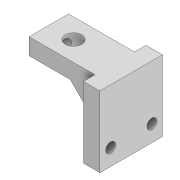
# Autodesk Inventor part: Mitutoyo holder
Saved by Autodesk Inventor 2020 (Build 240168000, 168)
## iProperties
Created: 2022-05-11
Part Number: Mitutoyo holder
Material: Generic
Document SubType Name: Modeling
Designer: ferrerx
Density: 1 g/cm^3
Appearance: Default
Author: ferrerx
Autodesk Inventor part; units mm, degrees
ref_plane "YZ Plane" through (0, 0, 0) normal (1, 0, 0) x (0, 1, 0)
ref_plane "XZ Plane" through (0, 0, 0) normal (0, 1, 0) x (-1, 0, 0)
ref_plane "XY Plane" through (0, 0, 0) normal (0, 0, 1) x (1, 0, 0)
sketch "Sketch1" plane through (0, 0, 0) normal (0, 1, 0) x (-1, 0, 0)
  circle A0 centre (19.9072, 0) radius 5
  line L0 (-15.0928, 12) -> (34.9072, 12)
  line L1 (34.9072, 12) -> (34.9072, -12)
  line L2 (34.9072, -12) -> (-15.0928, -12)
  line L3 (-15.0928, -12) -> (-15.0928, 12)
  point P0 (0, 0)
  dimension "d0" = 10
  dimension "d1" = 12
  dimension "d2" = 24
  dimension "d3" = 35
  dimension "d4" = 50
  constraints: 8 end point, 2 parallel, 1 centre point, 1 horizontal, 1 perpendicular
  measures "d0" diameter of A0
  measures "d1" distance from line of L0 A0.centre
  measures "d2" distance of L0.end L1.end
  measures "d3" distance from line of L3 A0.centre
  measures "d4" distance between parallel lines of L3 L1
extrude "Extrusion1" add sketch "Sketch1" along normal blind 10
sketch "Sketch2" plane through (15.0928, 0, 12) normal (1, 0, 0) x (0, 0, -1)
  line L0 (12, 0) -> (12, -23) construction
  line L1 (12, -23) -> (-0.5, -23) construction
  circle A0 centre (-0.5, -23) radius 3
  line L2 (31, 10) -> (-7, 10)
  line L3 (-7, 10) -> (-7, -33)
  line L4 (-7, -33) -> (31, -33)
  line L5 (31, -33) -> (31, 10)
  line L6 (31, 10) -> (-7, -33) construction
  line L7 (-7, 10) -> (31, -33) construction
  circle A1 centre (24.5, -23) radius 3
  point P0 (12, -11.5)
  dimension "d7" = 6
  dimension "d8" = 12.5
  constraints: 16 end point, 3 midpoint, 2 centre point, 2 horizontal, 2 parallel, 1 coincident, 1 perpendicular, 1 symmetric about line, 1 vertical, 1 other
  measures "d7" diameter of A0
  measures "d8" distance of L0.end L1.end
extrude "Extrusion2" add sketch "Sketch2" against normal blind 10
chamfer "Chamfer1" distance 15 angle 45 1 edges at (5.0928, 0, 0)
sketch "Sketch3" plane through (-34.9072, 0, -12) normal (-1, 0, 0) x (0, 0, 1)
  circle A0 centre (12, 5) radius 2.95
  line L0 (0, 10) -> (24, 10) projected
  point P0 (12, 0)
  dimension "d14" = 5.9
  dimension "d15" = 5
  constraints: 1 centre point
  measures "d14" diameter of A0
  measures "d15" distance from line of L0 A0.centre
extrude "Extrusion3" cut sketch "Sketch3" against normal blind 16
body "Solid1"
